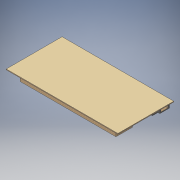
# Autodesk Inventor part: Foor
Saved by Autodesk Inventor 2018 (Build 220112000, 112)
## iProperties
Created: 2019-05-10
Part Number: Foor
Material: Generic
Document SubType Name: Modeling
Designer: 10043883
Density: 1 g/cm^3
Appearance: Natural Maple - Glossy Dark Tint
Author: 10043883
Autodesk Inventor part; units mm, degrees
ref_plane "YZ Plane" through (0, 0, 0) normal (1, 0, 0) x (0, 1, 0)
ref_plane "XZ Plane" through (0, 0, 0) normal (0, 1, 0) x (-1, 0, 0)
ref_plane "XY Plane" through (0, 0, 0) normal (0, 0, 1) x (1, 0, 0)
sketch "Sketch1" plane through (0, 0, 0) normal (0, 1, 0) x (-1, 0, 0)
  line L0 (3048, 1524) -> (-3048, 1524)
  line L1 (-3048, 1524) -> (-3048, -1524)
  line L2 (-3048, -1524) -> (3048, -1524)
  line L3 (3048, -1524) -> (3048, 1524)
  line L4 (3048, 1524) -> (-3048, -1524) construction
  line L5 (-3048, 1524) -> (3048, -1524) construction
  point P0 (0, 0)
  dimension "d0" = 6096
  dimension "d1" = 3048
  constraints: 12 end point, 2 midpoint, 2 parallel, 1 horizontal, 1 perpendicular
  measures "d0" distance of L2.end L1.end
  measures "d1" distance of L1.end L0.end
extrude "Extrusion1" add sketch "Sketch1" along normal blind 254
pattern_linear "Rectangular Pattern1" count 6 spacing 6096 along (1, 0, 0) count 6 spacing 3048 along (0, 0, -1) of "Extrusion1"
sketch "Sketch4" plane through (0, 0, 0) normal (0, -1, 0) x (1, 0, 0)
  line L0 (0, 0) -> (31365.9771, 0)
  line L1 (31365.9771, 0) -> (31365.9771, -5406.1685)
  line L2 (31365.9771, -5406.1685) -> (0, -5406.1685)
  line L3 (0, -5406.1685) -> (0, 0)
  line L4 (0, -11934.372) -> (4386.1366, -11934.372)
  line L5 (4386.1366, -11934.372) -> (4386.1366, -16167.5039)
  line L6 (4386.1366, -16167.5039) -> (0, -16167.5039)
  line L7 (0, -16167.5039) -> (0, -11934.372)
  line L8 (26418.823, -11934.372) -> (31365.9771, -11934.372)
  line L9 (31365.9771, -11934.372) -> (31365.9771, -16167.5039)
  line L10 (31365.9771, -16167.5039) -> (26418.823, -16167.5039)
  line L11 (26418.823, -16167.5039) -> (26418.823, -11934.372)
  constraints: 24 end point, 6 parallel, 4 point on line, 3 horizontal, 3 perpendicular
extrude "Extrusion4" add sketch "Sketch4" along normal blind 2540
sketch "Sketch5" plane through (4386.1366, 0, -16167.5039) normal (0, 0, -1) x (-1, 0, 0)
  line L0 (4080.5054, -2249.446) -> (302.9032, -2249.446)
  line L1 (302.9032, -2249.446) -> (302.9032, 0)
  line L2 (302.9032, 0) -> (4080.5054, 0)
  line L3 (4080.5054, 0) -> (4080.5054, -2249.446)
  point P0 (4386.1366, 0)
  constraints: 8 end point, 2 parallel, 1 horizontal, 1 perpendicular
sketch "Sketch6" plane through (0, 0, -16167.5039) normal (-1, 0, 0) x (0, 0, 1)
  line L0 (17691.5039, 0) -> (-596.4961, 0) projected
  line L1 (3978.2146, -2297.8832) -> (339.7137, -2297.8832)
  line L2 (339.7137, -2297.8832) -> (339.7137, 0)
  line L3 (339.7137, 0) -> (3978.2146, 0)
  line L4 (3978.2146, 0) -> (3978.2146, -2297.8832)
  point P0 (16167.5039, 0)
  constraints: 8 end point, 2 parallel, 1 horizontal, 1 perpendicular, 1 point on line
extrude "Extrusion5" cut sketch "Sketch6" against normal through all
extrude "Extrusion6" cut sketch "Sketch5" against normal blind 5080
sketch "Sketch7" plane through (31365.9771, 0, -16167.5039) normal (0, 0, -1) x (-1, 0, 0)
  line L0 (0, 0) -> (4947.1541, 0) projected
  line L1 (4947.1541, -2297.8832) -> (0, -2297.8832) projected
  line L2 (4721.2839, 0) -> (232.745, 0)
  line L3 (232.745, 0) -> (232.745, -2297.8832)
  line L4 (232.745, -2297.8832) -> (4721.2839, -2297.8832)
  line L5 (4721.2839, -2297.8832) -> (4721.2839, 0)
  point P0 (31365.9771, 0)
  constraints: 8 end point, 2 parallel, 2 point on line, 1 horizontal, 1 perpendicular
extrude "Extrusion7" cut sketch "Sketch7" against normal blind 5080
sketch "Sketch8" plane through (0, 0, 0) normal (0, -1, 0) x (1, 0, 0)
  line L0 (-2841.6696, -12477.9229) -> (-313.7412, -12477.9229)
  line L1 (-313.7412, -12477.9229) -> (-313.7412, -15914.3253)
  line L2 (-313.7412, -15914.3253) -> (-2841.6696, -15914.3253)
  line L3 (-2841.6696, -15914.3253) -> (-2841.6696, -12477.9229)
  line L4 (31759.3504, -12477.9229) -> (33260.3079, -12477.9229)
  line L5 (33260.3079, -12477.9229) -> (33260.3079, -15598.3343)
  line L6 (33260.3079, -15598.3343) -> (31759.3504, -15598.3343)
  line L7 (31759.3504, -15598.3343) -> (31759.3504, -12477.9229)
  line L8 (24017.5697, -12477.9229) -> (26150.5093, -12477.9229)
  line L9 (26150.5093, -12477.9229) -> (26150.5093, -15598.3343)
  line L10 (26150.5093, -15598.3343) -> (24017.5697, -15598.3343)
  line L11 (24017.5697, -15598.3343) -> (24017.5697, -12477.9229)
  line L12 (4742.1156, -12477.9229) -> (6756.5585, -12477.9229)
  line L13 (6756.5585, -12477.9229) -> (6756.5585, -15598.3343)
  line L14 (6756.5585, -15598.3343) -> (4742.1156, -15598.3343)
  line L15 (4742.1156, -15598.3343) -> (4742.1156, -12477.9229)
  point P0 (0, 0)
  constraints: 32 end point, 8 parallel, 4 horizontal, 4 perpendicular, 2 point on line
extrude "Extrusion8" add sketch "Sketch8" along normal blind 1270
sketch "Sketch9" plane through (6756.5585, 0, -12477.9229) normal (1, 0, 0) x (0, 0, -1)
  line L0 (0, 0) -> (3120.4114, 0) projected
  line L1 (2838.981, -1113.43) -> (262.7905, -1113.43)
  line L2 (262.7905, -1113.43) -> (262.7905, 0)
  line L3 (262.7905, 0) -> (2838.981, 0)
  line L4 (2838.981, 0) -> (2838.981, -1113.43)
  point P0 (-12477.9229, 0)
  constraints: 8 end point, 2 parallel, 1 horizontal, 1 perpendicular, 1 point on line
extrude "Extrusion9" cut sketch "Sketch9" against normal through all
sketch "Sketch10" plane through (33260.3079, 0, -12477.9229) normal (1, 0, 0) x (0, 0, -1)
  line L0 (3120.4114, 0) -> (0, 0) projected
  line L1 (2646.51, -975.381) -> (366.2523, -975.381)
  line L2 (366.2523, -975.381) -> (366.2523, 0)
  line L3 (366.2523, 0) -> (2646.51, 0)
  line L4 (2646.51, 0) -> (2646.51, -975.381)
  point P0 (-12477.9229, 0)
  constraints: 8 end point, 2 parallel, 1 horizontal, 1 perpendicular, 1 point on line
extrude "Extrusion10" cut sketch "Sketch10" against normal through all
sketch "Sketch11" plane through (31365.9771, 0, -5406.1685) normal (0, 0, -1) x (-1, 0, 0)
  point P0 (31365.9771, 0)
body "Solid1"
